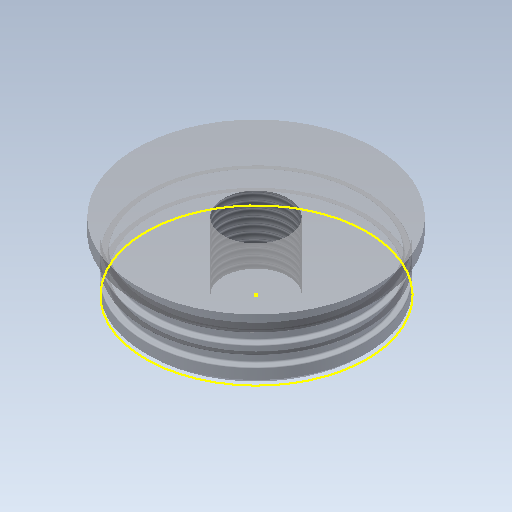
# Autodesk Inventor part: Deckel
Saved by Autodesk Inventor 2020.2 (Build 242310000, 310)
## iProperties
Created: 2014-03-26
Part Number: Deckel
Material: PMMA-Kunststoff
Document SubType Name: Modeling
Designer: demo.user
Density: 1.188 g/cm^3
Appearance: Polycarbonat - klar
Mass: 46.8632 g
Surface Area: 80.0202 cm^2
Volume: 39.4471 cm^3
Author: demo.user
Autodesk Inventor part; units mm, degrees
ref_plane "XZ Plane" through (0, 0, 0) normal (0, 1, 0) x (-1, 0, 0)
ref_plane "XY Plane" through (0, 0, 0) normal (0, 0, 1) x (1, 0, 0)
sketch "Skizze1" plane through (0, 0, 0) normal (0, 0, 1) x (1, 0, 0)
  circle A0 centre (0, 0) radius 26.5
  dimension "d0" = 53
  constraints: 1 centre point, 1 coincident
  measures "d0" diameter of A0
extrude "Extrusion1" add sketch "Skizze1" along normal blind 15
sketch "Skizze2" plane through (0, 0, 0) normal (0, 0, -1) x (-1, 0, 0)
  circle A0 centre (0, 0) radius 24.5
  circle A1 centre (0, 0) radius 26.5 projected
  dimension "d3" = 49
  constraints: 1 centre point, 1 coincident
  measures "d3" diameter of A0
extrude "Extrusion2" cut sketch "Skizze2" against normal blind 12
sketch "Skizze3" plane through (0, 0, 0) normal (0, 0, -1) x (-1, 0, 0)
  circle A0 centre (0, 0) radius 24.5 projected
ref_plane "Arbeitsebene1" through (0, 0, 0) normal (1, 0, 0) x (0, 1, 0)
sketch "Skizze4" plane through (0, 0, 0) normal (1, 0, 0) x (0, 1, 0)
  line L0 (26.5, 12) -> (-26.5, 12) projected
  line L1 (24.5, 0) -> (24.5, 12) projected
  line L2 (24.5, 10) -> (23.2, 10)
  line L3 (23.2, 10) -> (23.2, 7.7)
  line L4 (23.2, 7.7) -> (24.5, 7.7)
  line L5 (24.5, 5.7) -> (23.2, 5.7)
  line L6 (23.2, 5.7) -> (23.2, 3.4)
  line L7 (23.2, 3.4) -> (24.5, 3.4)
  line L8 (0, -2.4) -> (0, 14.4) projected
  point P0 (0, 0)
  dimension "t" = 1.3
  dimension "b" = 2.3
  dimension "a" = 2
  dimension "d10" = 2
  constraints: 12 end point, 5 perpendicular, 4 point on line, 2 equal length, 1 parallel
  measures "t" distance of L2.start L2.end
  measures "b" distance of L2.end L3.end
  measures "a" distance from line of L2 L1.end
  measures "d10" distance of L5.start L4.end
revolve "Umdrehung1" cut sketch "Skizze4" angle 360 about axis through (0, 0, -10) along (0, 0, 1)
chamfer "Fase1" distance 1 angle 45 1 edges at (24.5, 0, 0)
fillet "Rundung1" radius 0.2 4 edges at (24.5, 0, 3.4) (24.5, 0, 5.7) (24.5, 0, 7.7) (24.5, 0, 10)
fillet "Rundung1" radius 0.3 4 edges at (0, -23.2, 3.4) (0, -23.2, 5.7) (0, -23.2, 7.7) (0, -23.2, 10)
sketch "Skizze5" plane through (0, 0, 15) normal (0, 0, 1) x (1, 0, 0)
  circle A0 centre (0, 0) radius 26.5 projected
  constraints: 1 coincident
hole "Bohrung1" at (0, 0, 15) direction (0, 0, -1) diameter 14.376 end through all thread size "M16x1.5" class "6H" standard "ANSI Metric M Profile"
equation "\"d10\" = a"
